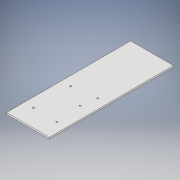
# Autodesk Inventor part: Cuerpo - Base
Saved by Autodesk Inventor 2019 (Build 230136000, 136)
## iProperties
Created: 2020-02-15
Part Number: Cuerpo - Base
Material: ABS Plastic
Document SubType Name: Modeling
Designer: Mafer1
Density: 1.06 g/cm^3
Appearance: Smooth - White
Mass: 43.8755 g
Surface Area: 296.565 cm^2
Volume: 41.392 cm^3
ancho_base: 100.000 mm
largo_base: 200.000 mm
Author: Mafer1
Autodesk Inventor part; units mm, degrees
ref_plane "YZ Plane" through (0, 0, 0) normal (1, 0, 0) x (0, 1, 0)
ref_plane "XZ Plane" through (0, 0, 0) normal (0, 1, 0) x (-1, 0, 0)
ref_plane "XY Plane" through (0, 0, 0) normal (0, 0, 1) x (1, 0, 0)
sketch "Boceto1" plane through (0, 0, 0) normal (0, 1, 0) x (-1, 0, 0)
  line L0 (0, 0) -> (86.188, 0)
  line L1 (86.188, 0) -> (86.188, -250)
  line L2 (86.188, -250) -> (0, -250)
  line L3 (0, -250) -> (0, 0)
  dimension "d0" = 250
  dimension "d1" = 86.188
  constraints: 8 end point, 2 parallel, 1 horizontal, 1 perpendicular
  measures "d0" distance of L0.end L1.end
  measures "d1" distance between parallel lines of L3 L1
extrude "Extrusión1" add sketch "Boceto1" along normal blind 3.3
sketch "Sketch3" plane through (0, 3.3, 0) normal (0, 1, 0) x (1, 0, 0)
  line L0 (-86.188, 250) -> (-86.188, 0) projected
  line L1 (-69.769, 121.59) -> (-16.419, 121.59) construction
  line L2 (-16.419, 121.59) -> (-16.419, 20) construction
  line L3 (-16.419, 20) -> (-69.769, 20) construction
  line L4 (-69.769, 20) -> (-69.769, 121.59) construction
  line L5 (0, 250) -> (-86.188, 250) projected
  circle A0 centre (-67.219, 35.24) radius 1.5875
  circle A1 centre (-18.959, 33.97) radius 1.5875
  circle A2 centre (-18.959, 116.52) radius 1.5875
  circle A3 centre (-67.219, 110.17) radius 1.5875
  circle A4 centre (-24.039, 86.04) radius 1.5875
  line L6 (-86.188, 0) -> (0, 0) projected
  dimension "d21" = 101.59
  dimension "d22" = 53.35
  dimension "d23" = 16.419
  dimension "d25" = 15.24
  dimension "d26" = 3.175
  dimension "d28" = 50.8
  dimension "d29" = 13.97
  dimension "d30" = 2.54
  dimension "d31" = 90.17
  dimension "d32" = 96.52
  dimension "d34" = 50.8
  dimension "d35" = 2.54
  dimension "d36" = 66.04
  dimension "d37" = 7.62
  dimension "d49" = 86.188
  dimension "d50" = 20
  constraints: 8 end point, 5 centre point, 4 equal radius, 2 parallel, 1 horizontal, 1 perpendicular
  measures "d21" distance of L1.end L2.end
  measures "d22" distance of L2.end L3.end
  measures "d23" distance between parallel lines of L4 L0
  measures "d25" distance from line of L3 A0.centre
  measures "d26" diameter of A0
  measures "d28" distance from line of A0.centre L2
  measures "d29" distance from line of L3 A1.centre
  measures "d30" distance from line of A1.centre L2
  measures "d31" distance from line of A3.centre L3
  measures "d32" distance from line of A2.centre L3
  measures "d34" distance from line of A3.centre L2
  measures "d35" distance from line of A2.centre L2
  measures "d36" distance from line of A4.centre L3
  measures "d37" distance from line of A4.centre L2
  measures "d49" distance of L5.start L0.start
  measures "d50" distance between parallel lines of L6 L3
extrude "Extrusion5" cut sketch "Sketch3" against normal up to surface (3.3 mm away)
equation "\"d1\" = ancho_acople_hombros"
equation "\"d23\" = -0.5 * d22 + 0.5 * d49"
equation "\"d34\" = d28"
equation "\"d35\" = d30"
equation "\"ancho_base\" = 100"
equation "\"ancho_acople_hombros\" = 86.188"
